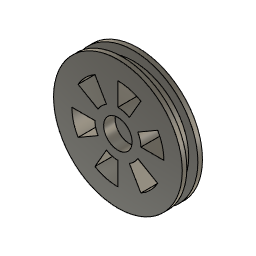
Wheel v8 (Autodesk Fusion 360 design; units mm, degrees)
Autodesk Fusion 360 part; units mm, degrees
note: some values were not read from the file. Set by a fixed rule: which sketch regions a step uses.
sketch "Sketch1" plane through (0, 0, 0) normal (1, 0, 0) x (0, 1, 0)
  line L0 (0, 14) -> (1, 14)
  line L1 (3.4, 14) -> (4.4, 14)
  line L2 (4.4, 14) -> (4.4, 0)
  line L3 (2.5, 0) -> (4.4, 0)
  line L4 (1, 14) -> (1, 12)
  line L5 (3.4, 14) -> (3.4, 12)
  line L6 (1, 12) -> (3.4, 12)
  line L7 (2.5, 0) -> (2.5, 3.1)
  line L8 (2.5, 3.1) -> (2.3751, 3.1)
  line L9 (2.3751, 3.1) -> (0, 3.1)
  line L10 (0, 14) -> (0, 3.1)
  dimension "d3" = 1
  dimension "d7" = 1
  dimension "d8" = 14
  dimension "d11" = 1.9
  dimension "d20" = 2
  dimension "d21" = 2
  dimension "d22" = 2.4
  dimension "d25" = 3.1
  constraint perpendicular L1 L2
  constraint perpendicular L2 L3
  constraint perpendicular L0 L4
  constraint perpendicular L1 L5
  constraint perpendicular L5 L6
  constraint perpendicular L3 L7
  constraint perpendicular L7 L8
  constraint perpendicular L7 L9
  constraint perpendicular L9 L10
  measures "d3" distance of L0.start L0.end
  measures "d7" distance of L1.start L1.end
  measures "d8" distance of L1.end L2.end
  measures "d11" distance of L3.start L2.end
  measures "d20" distance of L0.end L4.end
  measures "d21" distance of L1.start L5.end
  measures "d22" distance of L4.end L5.end
  measures "d25" distance of L3.start L7.end
revolve "Revolve1" add sketch "Sketch1" angle 360 about axis through (0, 1.75, 0) along (0, 1, 0)
sketch "Sketch2" plane through (0, 0, 0) normal (0, 1, 0) x (1, 0, 0)
  line L0 (5, 0) -> (10, 0)
  line L1 (4.3301, -2.5) -> (8.6603, -5)
  arc A0 (4.3301, -2.5) -> (5, 0) centre (0, 0) ccw
  arc A1 (8.6603, -5) -> (10, 0) centre (0, 0) ccw
  dimension "d13" = 30
  dimension "d14" = 20
  dimension "d15" = 10
  constraint horizontal L0
  constraint coincident A0.centre A1.centre
  constraint concentric A0 A1
  measures "d13" angle of L0 L1
  measures "d14" diameter of A1
  measures "d15" diameter of A0
extrude "Extrude1" cut sketch "Sketch2" along normal blind 5
pattern_circular "C-Pattern1" count 6 over 360 about axis through (0, 0, 0) along (0, 1, 0) of "Extrude1"
move_body "Move1" bodies 1 to x (1, 0, 0) y (0, 0, -1) z (0, 1, 0) at (0, 13, -11)
move_body "Move2" bodies 1 to x (1, 0, 0) y (0, 1, 0) z (0, 0, 1) at (0, 0, 15.4)
move_body "Move3" bodies 1 to x (1, 0, 0) y (0, 0, 1) z (0, -1, 0) at (0, 17.4, -8.6)
